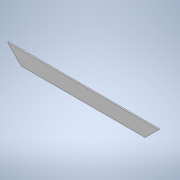
# Autodesk Inventor part: angle2
Saved by Autodesk Inventor 2020.1 (Build 241239000, 239)
## iProperties
Created: 2021-08-04
Part Number: angle2
Material: Generic
Document SubType Name: Modeling
Designer: Caleb
Density: 1 g/cm^3
Appearance: Default
Author: Caleb
Autodesk Inventor part; units mm, degrees
ref_plane "YZ Plane" through (0, 0, 0) normal (1, 0, 0) x (0, 1, 0)
ref_plane "XZ Plane" through (0, 0, 0) normal (0, 1, 0) x (-1, 0, 0)
ref_plane "XY Plane" through (0, 0, 0) normal (0, 0, 1) x (1, 0, 0)
sketch "Sketch1" plane through (0, 0, 0) normal (0, 1, 0) x (-1, 0, 0)
  line L0 (275, 24.5536) -> (-275, 24.5536)
  line L1 (-275, 24.5536) -> (-275, -24.5536)
  line L2 (-275, -24.5536) -> (275, -24.5536)
  line L3 (275, -24.5536) -> (275, 24.5536)
  point P0 (0, 0)
  dimension "d14" = 550
  constraints: 8 end point, 2 parallel, 1 horizontal, 1 perpendicular
  measures "d14" distance of L1.end L2.end
extrude "Extrusion1" add sketch "Sketch1" along normal mid plane 50
sketch "Sketch2" plane through (275, -25, -24.5536) normal (1, 0, 0) x (0, 0, -1)
  line L0 (0, 0) -> (0, 5)
  line L1 (0, 0) -> (0, 50) projected
  line L2 (0, 5) -> (-45, 5)
  line L3 (-45, 5) -> (-45, 50)
  line L4 (-49.1071, 50) -> (0, 50) projected
  line L5 (-45, 50) -> (0, 50)
  line L6 (0, 50) -> (0, 5)
  point P0 (-24.5536, 25)
  constraints: 10 end point, 3 perpendicular, 2 point on line, 1 horizontal
extrude "Extrusion2" cut sketch "Sketch2" against normal through all
sketch "Sketch5" plane through (0, -25, 0) normal (0, -1, 0) x (1, 0, 0)
  line L0 (275, 20.4464) -> (-275, 20.4464) projected
  line L1 (-275, -24.5536) -> (-275, 20.4464)
  line L2 (-275, 20.4464) -> (-225, 20.4464)
  line L3 (-225, 20.4464) -> (-225, -24.5536)
  line L4 (-225, -24.5536) -> (-275, -24.5536)
  line L5 (-275, -24.5536) -> (275, -24.5536) projected
  line L6 (275, -24.5536) -> (275, 20.4464)
  line L7 (275, -24.5536) -> (275, 24.5536) projected
  line L8 (275, 20.4464) -> (225, 20.4464)
  line L9 (225, 20.4464) -> (225, -24.5536)
  line L10 (225, -24.5536) -> (275, -24.5536)
  point P0 (0, 0)
  constraints: 16 end point, 5 perpendicular, 5 point on line
extrude "Extrusion5" cut sketch "Sketch5" against normal blind 10 contours L6 L5 L9 L0 | L3 L4 L1 L0
sketch "Sketch6" plane through (-275, 25, 24.5536) normal (0, 0, 1) x (1, 0, 0)
  line L0 (50, -50) -> (50, -45) projected
  line L1 (50, -50) -> (0, 0)
  line L2 (0, 0) -> (0, -50)
  line L3 (0, -50) -> (50, -50)
  line L4 (550, -50) -> (0, -50) projected
  line L5 (500, -50) -> (550, -50)
  line L6 (550, -50) -> (550, 0) projected
  line L7 (550, -50) -> (550, 0)
  line L8 (550, 0) -> (500, -50)
  point P0 (275, -25)
  constraints: 12 end point, 2 collinear, 2 perpendicular, 1 parallel
extrude "Extrusion6" cut sketch "Sketch6" against normal blind 5
body "Solid1"
